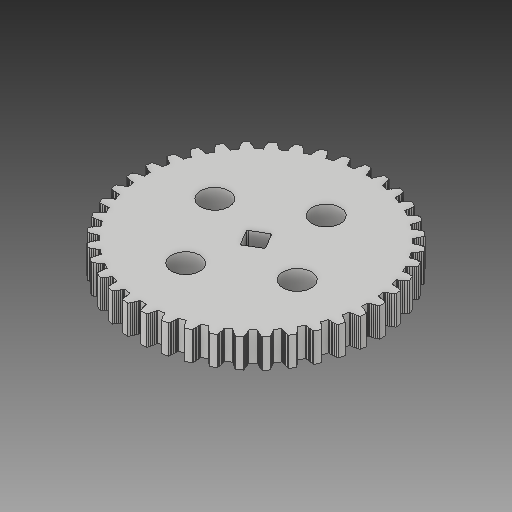
# Autodesk Inventor part: gear40
Saved by Autodesk Inventor 2019 (Build 230136000, 136)
## iProperties
Created: 2018-12-28
Part Number: gear40
Material: Generic
Document SubType Name: Modeling
Designer: Varga Daniel
Density: 1 g/cm^3
Appearance: Default
Sending System: SolidWorks 2018
Last Author: david
Last Saved: 2018-12-28
Author: Varga Daniel
Autodesk Inventor part; units mm, degrees
ref_plane "YZ Plane" through (0, 0, 0) normal (1, 0, 0) x (0, 1, 0)
ref_plane "XZ Plane" through (0, 0, 0) normal (0, 1, 0) x (-1, 0, 0)
ref_plane "XY Plane" through (0, 0, 0) normal (0, 0, 1) x (1, 0, 0)
sketch "Sketch5" plane through (0, 0, 0) normal (0, 1, 0) x (-1, 0, 0)
  line L0 (1.6245, 18.6336) -> (1.5605, 18.6409)
  line L1 (1.5605, 18.6409) -> (1.4964, 18.6492)
  line L2 (1.4964, 18.6492) -> (1.3679, 18.6686)
  line L3 (1.3679, 18.6686) -> (1.1102, 18.7172)
  line L4 (1.1102, 18.7172) -> (0.8515, 18.7777)
  line L5 (0.8515, 18.7777) -> (0.5922, 18.8492)
  line L6 (0.5922, 18.8492) -> (0.3324, 18.931)
  line L7 (0.3324, 18.931) -> (0.0723, 19.0226)
  line L8 (0.0723, 19.0226) -> (0.0134, 20.0093)
  line L9 (0.0134, 20.0093) -> (0.2607, 20.1312)
  line L10 (0.2607, 20.1312) -> (0.5089, 20.2434)
  line L11 (0.5089, 20.2434) -> (0.7578, 20.3453)
  line L12 (0.7578, 20.3453) -> (1.0074, 20.4362)
  line L13 (1.0074, 20.4362) -> (1.2576, 20.5151)
  line L14 (1.2576, 20.5151) -> (1.3828, 20.5496)
  line L15 (1.3828, 20.5496) -> (1.4455, 20.5655)
  line L16 (1.4455, 20.5655) -> (1.5081, 20.5804)
  line L17 (1.5081, 20.5804) -> (1.5283, 21.6521)
  line L18 (1.5283, 21.6521) -> (1.4663, 21.6694)
  line L19 (1.4663, 21.6694) -> (1.4042, 21.6877)
  line L20 (1.4042, 21.6877) -> (1.2804, 21.7268)
  line L21 (1.2804, 21.7268) -> (1.0334, 21.8151)
  line L22 (1.0334, 21.8151) -> (0.7874, 21.9154)
  line L23 (0.7874, 21.9154) -> (0.5425, 22.0266)
  line L24 (0.5425, 22.0266) -> (0.2987, 22.1481)
  line L25 (0.2987, 22.1481) -> (0.0561, 22.2792)
  line L26 (0.0561, 22.2792) -> (0.1523, 23.263)
  line L27 (0.1523, 23.263) -> (0.4156, 23.3447)
  line L28 (0.4156, 23.3447) -> (0.6783, 23.4167)
  line L29 (0.6783, 23.4167) -> (0.9401, 23.4783)
  line L30 (0.9401, 23.4783) -> (1.2009, 23.5291)
  line L31 (1.2009, 23.5291) -> (1.4603, 23.5679)
  line L32 (1.4603, 23.5679) -> (1.5894, 23.5824)
  line L33 (1.5894, 23.5824) -> (1.6537, 23.5883)
  line L34 (1.6537, 23.5883) -> (1.718, 23.5932)
  line L35 (1.718, 23.5932) -> (1.9056, 24.6486)
  line L36 (1.9056, 24.6486) -> (1.847, 24.6754)
  line L37 (1.847, 24.6754) -> (1.7886, 24.7031)
  line L38 (1.7886, 24.7031) -> (1.6724, 24.7612)
  line L39 (1.6724, 24.7612) -> (1.4423, 24.887)
  line L40 (1.4423, 24.887) -> (1.215, 25.0245)
  line L41 (1.215, 25.0245) -> (0.9905, 25.1727)
  line L42 (0.9905, 25.1727) -> (0.7687, 25.3308)
  line L43 (0.7687, 25.3308) -> (0.5496, 25.4982)
  line L44 (0.5496, 25.4982) -> (0.7984, 26.4549)
  line L45 (0.7984, 26.4549) -> (1.0713, 26.4944)
  line L46 (1.0713, 26.4944) -> (1.342, 26.5244)
  line L47 (1.342, 26.5244) -> (1.6103, 26.5443)
  line L48 (1.6103, 26.5443) -> (1.8758, 26.5537)
  line L49 (1.8758, 26.5537) -> (2.1381, 26.5514)
  line L50 (2.1381, 26.5514) -> (2.2678, 26.5455)
  line L51 (2.2678, 26.5455) -> (2.3323, 26.5413)
  line L52 (2.3323, 26.5413) -> (2.3965, 26.5361)
  line L53 (2.3965, 26.5361) -> (2.7469, 27.5491)
  line L54 (2.7469, 27.5491) -> (2.6932, 27.5847)
  line L55 (2.6932, 27.5847) -> (2.6399, 27.6213)
  line L56 (2.6399, 27.6213) -> (2.5342, 27.6968)
  line L57 (2.5342, 27.6968) -> (2.3266, 27.8571)
  line L58 (2.3266, 27.8571) -> (2.1237, 28.0284)
  line L59 (2.1237, 28.0284) -> (1.9251, 28.2099)
  line L60 (1.9251, 28.2099) -> (1.7307, 28.4007)
  line L61 (1.7307, 28.4007) -> (1.5406, 28.6004)
  line L62 (1.5406, 28.6004) -> (1.936, 29.5064)
  line L63 (1.936, 29.5064) -> (2.2117, 29.5027)
  line L64 (2.2117, 29.5027) -> (2.4838, 29.49)
  line L65 (2.4838, 29.49) -> (2.7519, 29.4677)
  line L66 (2.7519, 29.4677) -> (3.0155, 29.4354)
  line L67 (3.0155, 29.4354) -> (3.2742, 29.3922)
  line L68 (3.2742, 29.3922) -> (3.4015, 29.3661)
  line L69 (3.4015, 29.3661) -> (3.4645, 29.3518)
  line L70 (3.4645, 29.3518) -> (3.5271, 29.3366)
  line L71 (3.5271, 29.3366) -> (4.0316, 30.2823)
  line L72 (4.0316, 30.2823) -> (3.9842, 30.3259)
  line L73 (3.9842, 30.3259) -> (3.9372, 30.3703)
  line L74 (3.9372, 30.3703) -> (3.8447, 30.4614)
  line L75 (3.8447, 30.4614) -> (3.6647, 30.6522)
  line L76 (3.6647, 30.6522) -> (3.491, 30.8533)
  line L77 (3.491, 30.8533) -> (3.3233, 31.0636)
  line L78 (3.3233, 31.0636) -> (3.1612, 31.2824)
  line L79 (3.1612, 31.2824) -> (3.0046, 31.5094)
  line L80 (3.0046, 31.5094) -> (3.5369, 32.3423)
  line L81 (3.5369, 32.3423) -> (3.8086, 32.2956)
  line L82 (3.8086, 32.2956) -> (4.0754, 32.2404)
  line L83 (4.0754, 32.2404) -> (4.3367, 32.1765)
  line L84 (4.3367, 32.1765) -> (4.592, 32.1034)
  line L85 (4.592, 32.1034) -> (4.8408, 32.0202)
  line L86 (4.8408, 32.0202) -> (4.9624, 31.9745)
  line L87 (4.9624, 31.9745) -> (5.0224, 31.9505)
  line L88 (5.0224, 31.9505) -> (5.0819, 31.9258)
  line L89 (5.0819, 31.9258) -> (5.7281, 32.7809)
  line L90 (5.7281, 32.7809) -> (5.6881, 32.8314)
  line L91 (5.6881, 32.8314) -> (5.6487, 32.8826)
  line L92 (5.6487, 32.8826) -> (5.5715, 32.9871)
  line L93 (5.5715, 32.9871) -> (5.4236, 33.2037)
  line L94 (5.4236, 33.2037) -> (5.2835, 33.4294)
  line L95 (5.2835, 33.4294) -> (5.1507, 33.6633)
  line L96 (5.1507, 33.6633) -> (5.0248, 33.9049)
  line L97 (5.0248, 33.9049) -> (4.9057, 34.1535)
  line L98 (4.9057, 34.1535) -> (5.5617, 34.893)
  line L99 (5.5617, 34.893) -> (5.8228, 34.8043)
  line L100 (5.8228, 34.8043) -> (6.0776, 34.7081)
  line L101 (6.0776, 34.7081) -> (6.3257, 34.6041)
  line L102 (6.3257, 34.6041) -> (6.5665, 34.4919)
  line L103 (6.5665, 34.4919) -> (6.7992, 34.3708)
  line L104 (6.7992, 34.3708) -> (6.9121, 34.3067)
  line L105 (6.9121, 34.3067) -> (6.9677, 34.2736)
  line L106 (6.9677, 34.2736) -> (7.0225, 34.2398)
  line L107 (7.0225, 34.2398) -> (7.7946, 34.9834)
  line L108 (7.7946, 34.9834) -> (7.7629, 35.0395)
  line L109 (7.7629, 35.0395) -> (7.732, 35.0962)
  line L110 (7.732, 35.0962) -> (7.6721, 35.2115)
  line L111 (7.6721, 35.2115) -> (7.5599, 35.4486)
  line L112 (7.5599, 35.4486) -> (7.4569, 35.6934)
  line L113 (7.4569, 35.6934) -> (7.3623, 35.9452)
  line L114 (7.3623, 35.9452) -> (7.2758, 36.2035)
  line L115 (7.2758, 36.2035) -> (7.197, 36.4677)
  line L116 (7.197, 36.4677) -> (7.9606, 37.0954)
  line L117 (7.9606, 37.0954) -> (8.2046, 36.967)
  line L118 (8.2046, 36.967) -> (8.4412, 36.8321)
  line L119 (8.4412, 36.8321) -> (8.67, 36.6906)
  line L120 (8.67, 36.6906) -> (8.8903, 36.5421)
  line L121 (8.8903, 36.5421) -> (9.1012, 36.3861)
  line L122 (9.1012, 36.3861) -> (9.2027, 36.3051)
  line L123 (9.2027, 36.3051) -> (9.2524, 36.2638)
  line L124 (9.2524, 36.2638) -> (9.3013, 36.2218)
  line L125 (9.3013, 36.2218) -> (10.1802, 36.8354)
  line L126 (10.1802, 36.8354) -> (10.1577, 36.8958)
  line L127 (10.1577, 36.8958) -> (10.136, 36.9567)
  line L128 (10.136, 36.9567) -> (10.0949, 37.0799)
  line L129 (10.0949, 37.0799) -> (10.0212, 37.3316)
  line L130 (10.0212, 37.3316) -> (9.9577, 37.5896)
  line L131 (9.9577, 37.5896) -> (9.9037, 37.8531)
  line L132 (9.9037, 37.8531) -> (9.8586, 38.1217)
  line L133 (9.8586, 38.1217) -> (9.8221, 38.395)
  line L134 (9.8221, 38.395) -> (10.6746, 38.8955)
  line L135 (10.6746, 38.8955) -> (10.8954, 38.7305)
  line L136 (10.8954, 38.7305) -> (11.1081, 38.5603)
  line L137 (11.1081, 38.5603) -> (11.3119, 38.3847)
  line L138 (11.3119, 38.3847) -> (11.5062, 38.2036)
  line L139 (11.5062, 38.2036) -> (11.6901, 38.0165)
  line L140 (11.6901, 38.0165) -> (11.7777, 37.9206)
  line L141 (11.7777, 37.9206) -> (11.8203, 37.872)
  line L142 (11.8203, 37.872) -> (11.862, 37.823)
  line L143 (11.862, 37.823) -> (12.8261, 38.2915)
  line L144 (12.8261, 38.2915) -> (12.8133, 38.3546)
  line L145 (12.8133, 38.3546) -> (12.8014, 38.4182)
  line L146 (12.8014, 38.4182) -> (12.7801, 38.5463)
  line L147 (12.7801, 38.5463) -> (12.7467, 38.8064)
  line L148 (12.7467, 38.8064) -> (12.7243, 39.0711)
  line L149 (12.7243, 39.0711) -> (12.7122, 39.3399)
  line L150 (12.7122, 39.3399) -> (12.7097, 39.6122)
  line L151 (12.7097, 39.6122) -> (12.7164, 39.8879)
  line L152 (12.7164, 39.8879) -> (13.6367, 40.2489)
  line L153 (13.6367, 40.2489) -> (13.829, 40.0513)
  line L154 (13.829, 40.0513) -> (14.0124, 39.8499)
  line L155 (14.0124, 39.8499) -> (14.1862, 39.6447)
  line L156 (14.1862, 39.6447) -> (14.3498, 39.4354)
  line L157 (14.3498, 39.4354) -> (14.5022, 39.2219)
  line L158 (14.5022, 39.2219) -> (14.5737, 39.1134)
  line L159 (14.5737, 39.1134) -> (14.6082, 39.0587)
  line L160 (14.6082, 39.0587) -> (14.6417, 39.0038)
  line L161 (14.6417, 39.0038) -> (15.6672, 39.3157)
  line L162 (15.6672, 39.3157) -> (15.6645, 39.3801)
  line L163 (15.6645, 39.3801) -> (15.6627, 39.4447)
  line L164 (15.6627, 39.4447) -> (15.6617, 39.5746)
  line L165 (15.6617, 39.5746) -> (15.6693, 39.8368)
  line L166 (15.6693, 39.8368) -> (15.6886, 40.1017)
  line L167 (15.6886, 40.1017) -> (15.7187, 40.369)
  line L168 (15.7187, 40.369) -> (15.7589, 40.6384)
  line L169 (15.7589, 40.6384) -> (15.8086, 40.9096)
  line L170 (15.8086, 40.9096) -> (16.774, 41.1222)
  line L171 (16.774, 41.1222) -> (16.9331, 40.897)
  line L172 (16.9331, 40.897) -> (17.0827, 40.6694)
  line L173 (17.0827, 40.6694) -> (17.2223, 40.4394)
  line L174 (17.2223, 40.4394) -> (17.3511, 40.2071)
  line L175 (17.3511, 40.2071) -> (17.4682, 39.9724)
  line L176 (17.4682, 39.9724) -> (17.5219, 39.8541)
  line L177 (17.5219, 39.8541) -> (17.5474, 39.7948)
  line L178 (17.5474, 39.7948) -> (17.5719, 39.7352)
  line L179 (17.5719, 39.7352) -> (18.6336, 39.8829)
  line L180 (18.6336, 39.8829) -> (18.6409, 39.9469)
  line L181 (18.6409, 39.9469) -> (18.6493, 40.011)
  line L182 (18.6493, 40.011) -> (18.6686, 40.1394)
  line L183 (18.6686, 40.1394) -> (18.7172, 40.3972)
  line L184 (18.7172, 40.3972) -> (18.7777, 40.6558)
  line L185 (18.7777, 40.6558) -> (18.8492, 40.9152)
  line L186 (18.8492, 40.9152) -> (18.931, 41.175)
  line L187 (18.931, 41.175) -> (19.0226, 41.435)
  line L188 (19.0226, 41.435) -> (20.0093, 41.494)
  line L189 (20.0093, 41.494) -> (20.1312, 41.2467)
  line L190 (20.1312, 41.2467) -> (20.2434, 40.9985)
  line L191 (20.2434, 40.9985) -> (20.3453, 40.7495)
  line L192 (20.3453, 40.7495) -> (20.4362, 40.4999)
  line L193 (20.4362, 40.4999) -> (20.5151, 40.2498)
  line L194 (20.5151, 40.2498) -> (20.5496, 40.1246)
  line L195 (20.5496, 40.1246) -> (20.5655, 40.0619)
  line L196 (20.5655, 40.0619) -> (20.5804, 39.9993)
  line L197 (20.5804, 39.9993) -> (21.6521, 39.9791)
  line L198 (21.6521, 39.9791) -> (21.6694, 40.0411)
  line L199 (21.6694, 40.0411) -> (21.6877, 40.1031)
  line L200 (21.6877, 40.1031) -> (21.7269, 40.227)
  line L201 (21.7269, 40.227) -> (21.8151, 40.4739)
  line L202 (21.8151, 40.4739) -> (21.9154, 40.7199)
  line L203 (21.9154, 40.7199) -> (22.0266, 40.9649)
  line L204 (22.0266, 40.9649) -> (22.148, 41.2087)
  line L205 (22.148, 41.2087) -> (22.2792, 41.4512)
  line L206 (22.2792, 41.4512) -> (23.263, 41.3551)
  line L207 (23.263, 41.3551) -> (23.3447, 41.0918)
  line L208 (23.3447, 41.0918) -> (23.4167, 40.8291)
  line L209 (23.4167, 40.8291) -> (23.4783, 40.5672)
  line L210 (23.4783, 40.5672) -> (23.5291, 40.3065)
  line L211 (23.5291, 40.3065) -> (23.5679, 40.0471)
  line L212 (23.5679, 40.0471) -> (23.5824, 39.918)
  line L213 (23.5824, 39.918) -> (23.5883, 39.8536)
  line L214 (23.5883, 39.8536) -> (23.5932, 39.7894)
  line L215 (23.5932, 39.7894) -> (24.6486, 39.6018)
  line L216 (24.6486, 39.6018) -> (24.6754, 39.6604)
  line L217 (24.6754, 39.6604) -> (24.7031, 39.7188)
  line L218 (24.7031, 39.7188) -> (24.7612, 39.8349)
  line L219 (24.7612, 39.8349) -> (24.887, 40.0651)
  line L220 (24.887, 40.0651) -> (25.0245, 40.2924)
  line L221 (25.0245, 40.2924) -> (25.1727, 40.5169)
  line L222 (25.1727, 40.5169) -> (25.3307, 40.7387)
  line L223 (25.3307, 40.7387) -> (25.4982, 40.9577)
  line L224 (25.4982, 40.9577) -> (26.4549, 40.7089)
  line L225 (26.4549, 40.7089) -> (26.4944, 40.436)
  line L226 (26.4944, 40.436) -> (26.5243, 40.1653)
  line L227 (26.5243, 40.1653) -> (26.5443, 39.8971)
  line L228 (26.5443, 39.8971) -> (26.5537, 39.6316)
  line L229 (26.5537, 39.6316) -> (26.5514, 39.3693)
  line L230 (26.5514, 39.3693) -> (26.5455, 39.2395)
  line L231 (26.5455, 39.2395) -> (26.5413, 39.175)
  line L232 (26.5413, 39.175) -> (26.5361, 39.1108)
  line L233 (26.5361, 39.1108) -> (27.5491, 38.7604)
  line L234 (27.5491, 38.7604) -> (27.5847, 38.8141)
  line L235 (27.5847, 38.8141) -> (27.6212, 38.8675)
  line L236 (27.6212, 38.8675) -> (27.6968, 38.9731)
  line L237 (27.6968, 38.9731) -> (27.8571, 39.1807)
  line L238 (27.8571, 39.1807) -> (28.0284, 39.3837)
  line L239 (28.0284, 39.3837) -> (28.2099, 39.5823)
  line L240 (28.2099, 39.5823) -> (28.4007, 39.7766)
  line L241 (28.4007, 39.7766) -> (28.6004, 39.9668)
  line L242 (28.6004, 39.9668) -> (29.5064, 39.5714)
  line L243 (29.5064, 39.5714) -> (29.5027, 39.2957)
  line L244 (29.5027, 39.2957) -> (29.4899, 39.0236)
  line L245 (29.4899, 39.0236) -> (29.4677, 38.7555)
  line L246 (29.4677, 38.7555) -> (29.4354, 38.4918)
  line L247 (29.4354, 38.4918) -> (29.3922, 38.2331)
  line L248 (29.3922, 38.2331) -> (29.366, 38.1059)
  line L249 (29.366, 38.1059) -> (29.3518, 38.0429)
  line L250 (29.3518, 38.0429) -> (29.3366, 37.9802)
  line L251 (29.3366, 37.9802) -> (30.2823, 37.4757)
  line L252 (30.2823, 37.4757) -> (30.3259, 37.5231)
  line L253 (30.3259, 37.5231) -> (30.3704, 37.5702)
  line L254 (30.3704, 37.5702) -> (30.4615, 37.6628)
  line L255 (30.4615, 37.6628) -> (30.6523, 37.8427)
  line L256 (30.6523, 37.8427) -> (30.8533, 38.0164)
  line L257 (30.8533, 38.0164) -> (31.0636, 38.1842)
  line L258 (31.0636, 38.1842) -> (31.2825, 38.3463)
  line L259 (31.2825, 38.3463) -> (31.5095, 38.5028)
  line L260 (31.5095, 38.5028) -> (32.3424, 37.9706)
  line L261 (32.3424, 37.9706) -> (32.2956, 37.6988)
  line L262 (32.2956, 37.6988) -> (32.2405, 37.4321)
  line L263 (32.2405, 37.4321) -> (32.1766, 37.1708)
  line L264 (32.1766, 37.1708) -> (32.1035, 36.9154)
  line L265 (32.1035, 36.9154) -> (32.0203, 36.6667)
  line L266 (32.0203, 36.6667) -> (31.9746, 36.5451)
  line L267 (31.9746, 36.5451) -> (31.9506, 36.4851)
  line L268 (31.9506, 36.4851) -> (31.9259, 36.4256)
  line L269 (31.9259, 36.4256) -> (32.781, 35.7793)
  line L270 (32.781, 35.7793) -> (32.8315, 35.8194)
  line L271 (32.8315, 35.8194) -> (32.8827, 35.8588)
  line L272 (32.8827, 35.8588) -> (32.9872, 35.936)
  line L273 (32.9872, 35.936) -> (33.2038, 36.0839)
  line L274 (33.2038, 36.0839) -> (33.4295, 36.224)
  line L275 (33.4295, 36.224) -> (33.6634, 36.3567)
  line L276 (33.6634, 36.3567) -> (33.905, 36.4826)
  line L277 (33.905, 36.4826) -> (34.1536, 36.6018)
  line L278 (34.1536, 36.6018) -> (34.893, 35.9457)
  line L279 (34.893, 35.9457) -> (34.8044, 35.6847)
  line L280 (34.8044, 35.6847) -> (34.7082, 35.4298)
  line L281 (34.7082, 35.4298) -> (34.6042, 35.1817)
  line L282 (34.6042, 35.1817) -> (34.492, 34.941)
  line L283 (34.492, 34.941) -> (34.3709, 34.7083)
  line L284 (34.3709, 34.7083) -> (34.3067, 34.5953)
  line L285 (34.3067, 34.5953) -> (34.2737, 34.5398)
  line L286 (34.2737, 34.5398) -> (34.2399, 34.4849)
  line L287 (34.2399, 34.4849) -> (34.9834, 33.7128)
  line L288 (34.9834, 33.7128) -> (35.0395, 33.7445)
  line L289 (35.0395, 33.7445) -> (35.0963, 33.7754)
  line L290 (35.0963, 33.7754) -> (35.2116, 33.8353)
  line L291 (35.2116, 33.8353) -> (35.4486, 33.9475)
  line L292 (35.4486, 33.9475) -> (35.6935, 34.0506)
  line L293 (35.6935, 34.0506) -> (35.9453, 34.1451)
  line L294 (35.9453, 34.1451) -> (36.2036, 34.2316)
  line L295 (36.2036, 34.2316) -> (36.4678, 34.3104)
  line L296 (36.4678, 34.3104) -> (37.0955, 33.5468)
  line L297 (37.0955, 33.5468) -> (36.9671, 33.3028)
  line L298 (36.9671, 33.3028) -> (36.8322, 33.0662)
  line L299 (36.8322, 33.0662) -> (36.6907, 32.8374)
  line L300 (36.6907, 32.8374) -> (36.5422, 32.6171)
  line L301 (36.5422, 32.6171) -> (36.3862, 32.4063)
  line L302 (36.3862, 32.4063) -> (36.3052, 32.3048)
  line L303 (36.3052, 32.3048) -> (36.2638, 32.2551)
  line L304 (36.2638, 32.2551) -> (36.2219, 32.2062)
  line L305 (36.2219, 32.2062) -> (36.8355, 31.3273)
  line L306 (36.8355, 31.3273) -> (36.8959, 31.3498)
  line L307 (36.8959, 31.3498) -> (36.9568, 31.3715)
  line L308 (36.9568, 31.3715) -> (37.08, 31.4125)
  line L309 (37.08, 31.4125) -> (37.3317, 31.4863)
  line L310 (37.3317, 31.4863) -> (37.5896, 31.5498)
  line L311 (37.5896, 31.5498) -> (37.8532, 31.6038)
  line L312 (37.8532, 31.6038) -> (38.1218, 31.6488)
  line L313 (38.1218, 31.6488) -> (38.3951, 31.6853)
  line L314 (38.3951, 31.6853) -> (38.8956, 30.8329)
  line L315 (38.8956, 30.8329) -> (38.7306, 30.612)
  line L316 (38.7306, 30.612) -> (38.5603, 30.3994)
  line L317 (38.5603, 30.3994) -> (38.3848, 30.1956)
  line L318 (38.3848, 30.1956) -> (38.2037, 30.0012)
  line L319 (38.2037, 30.0012) -> (38.0166, 29.8174)
  line L320 (38.0166, 29.8174) -> (37.9207, 29.7298)
  line L321 (37.9207, 29.7298) -> (37.8721, 29.6872)
  line L322 (37.8721, 29.6872) -> (37.823, 29.6454)
  line L323 (37.823, 29.6454) -> (38.2916, 28.6814)
  line L324 (38.2916, 28.6814) -> (38.3547, 28.6941)
  line L325 (38.3547, 28.6941) -> (38.4183, 28.706)
  line L326 (38.4183, 28.706) -> (38.5464, 28.7273)
  line L327 (38.5464, 28.7273) -> (38.8065, 28.7608)
  line L328 (38.8065, 28.7608) -> (39.0712, 28.7831)
  line L329 (39.0712, 28.7831) -> (39.34, 28.7953)
  line L330 (39.34, 28.7953) -> (39.6123, 28.7977)
  line L331 (39.6123, 28.7977) -> (39.888, 28.791)
  line L332 (39.888, 28.791) -> (40.249, 27.8708)
  line L333 (40.249, 27.8708) -> (40.0514, 27.6784)
  line L334 (40.0514, 27.6784) -> (39.85, 27.4951)
  line L335 (39.85, 27.4951) -> (39.6447, 27.3212)
  line L336 (39.6447, 27.3212) -> (39.4354, 27.1576)
  line L337 (39.4354, 27.1576) -> (39.2219, 27.0053)
  line L338 (39.2219, 27.0053) -> (39.1135, 26.9338)
  line L339 (39.1135, 26.9338) -> (39.0588, 26.8993)
  line L340 (39.0588, 26.8993) -> (39.0038, 26.8657)
  line L341 (39.0038, 26.8657) -> (39.3158, 25.8402)
  line L342 (39.3158, 25.8402) -> (39.3802, 25.843)
  line L343 (39.3802, 25.843) -> (39.4448, 25.8448)
  line L344 (39.4448, 25.8448) -> (39.5747, 25.8458)
  line L345 (39.5747, 25.8458) -> (39.8368, 25.8382)
  line L346 (39.8368, 25.8382) -> (40.1018, 25.8188)
  line L347 (40.1018, 25.8188) -> (40.3691, 25.7887)
  line L348 (40.3691, 25.7887) -> (40.6385, 25.7486)
  line L349 (40.6385, 25.7486) -> (40.9097, 25.6988)
  line L350 (40.9097, 25.6988) -> (41.1223, 24.7334)
  line L351 (41.1223, 24.7334) -> (40.897, 24.5742)
  line L352 (40.897, 24.5742) -> (40.6693, 24.4246)
  line L353 (40.6693, 24.4246) -> (40.4394, 24.285)
  line L354 (40.4394, 24.285) -> (40.2071, 24.1561)
  line L355 (40.2071, 24.1561) -> (39.9723, 24.0391)
  line L356 (39.9723, 24.0391) -> (39.8541, 23.9854)
  line L357 (39.8541, 23.9854) -> (39.7947, 23.9599)
  line L358 (39.7947, 23.9599) -> (39.7351, 23.9354)
  line L359 (39.7351, 23.9354) -> (39.8828, 22.8737)
  line L360 (39.8828, 22.8737) -> (39.9468, 22.8664)
  line L361 (39.9468, 22.8664) -> (40.0109, 22.858)
  line L362 (40.0109, 22.858) -> (40.1393, 22.8387)
  line L363 (40.1393, 22.8387) -> (40.3971, 22.7901)
  line L364 (40.3971, 22.7901) -> (40.6558, 22.7296)
  line L365 (40.6558, 22.7296) -> (40.9151, 22.6581)
  line L366 (40.9151, 22.6581) -> (41.1749, 22.5763)
  line L367 (41.1749, 22.5763) -> (41.435, 22.4847)
  line L368 (41.435, 22.4847) -> (41.4939, 21.498)
  line L369 (41.4939, 21.498) -> (41.2466, 21.3761)
  line L370 (41.2466, 21.3761) -> (40.9984, 21.2639)
  line L371 (40.9984, 21.2639) -> (40.7494, 21.162)
  line L372 (40.7494, 21.162) -> (40.4998, 21.0711)
  line L373 (40.4998, 21.0711) -> (40.2497, 20.9922)
  line L374 (40.2497, 20.9922) -> (40.1245, 20.9577)
  line L375 (40.1245, 20.9577) -> (40.0618, 20.9418)
  line L376 (40.0618, 20.9418) -> (39.9991, 20.9268)
  line L377 (39.9991, 20.9268) -> (39.9789, 19.8552)
  line L378 (39.9789, 19.8552) -> (40.041, 19.8379)
  line L379 (40.041, 19.8379) -> (40.103, 19.8196)
  line L380 (40.103, 19.8196) -> (40.2268, 19.7804)
  line L381 (40.2268, 19.7804) -> (40.4738, 19.6922)
  line L382 (40.4738, 19.6922) -> (40.7198, 19.5919)
  line L383 (40.7198, 19.5919) -> (40.9647, 19.4807)
  line L384 (40.9647, 19.4807) -> (41.2085, 19.3592)
  line L385 (41.2085, 19.3592) -> (41.4511, 19.2281)
  line L386 (41.4511, 19.2281) -> (41.355, 18.2443)
  line L387 (41.355, 18.2443) -> (41.0918, 18.1626)
  line L388 (41.0918, 18.1626) -> (40.8291, 18.0907)
  line L389 (40.8291, 18.0907) -> (40.5673, 18.029)
  line L390 (40.5673, 18.029) -> (40.3066, 17.9782)
  line L391 (40.3066, 17.9782) -> (40.0472, 17.9394)
  line L392 (40.0472, 17.9394) -> (39.9181, 17.9249)
  line L393 (39.9181, 17.9249) -> (39.8537, 17.919)
  line L394 (39.8537, 17.919) -> (39.7895, 17.9141)
  line L395 (39.7895, 17.9141) -> (39.6018, 16.8587)
  line L396 (39.6018, 16.8587) -> (39.6604, 16.832)
  line L397 (39.6604, 16.832) -> (39.7188, 16.8042)
  line L398 (39.7188, 16.8042) -> (39.835, 16.7462)
  line L399 (39.835, 16.7462) -> (40.0651, 16.6203)
  line L400 (40.0651, 16.6203) -> (40.2924, 16.4828)
  line L401 (40.2924, 16.4828) -> (40.517, 16.3346)
  line L402 (40.517, 16.3346) -> (40.7388, 16.1766)
  line L403 (40.7388, 16.1766) -> (40.9578, 16.0091)
  line L404 (40.9578, 16.0091) -> (40.709, 15.0524)
  line L405 (40.709, 15.0524) -> (40.4361, 15.0129)
  line L406 (40.4361, 15.0129) -> (40.1654, 14.983)
  line L407 (40.1654, 14.983) -> (39.8971, 14.963)
  line L408 (39.8971, 14.963) -> (39.6316, 14.9536)
  line L409 (39.6316, 14.9536) -> (39.3694, 14.9559)
  line L410 (39.3694, 14.9559) -> (39.2396, 14.9618)
  line L411 (39.2396, 14.9618) -> (39.1751, 14.966)
  line L412 (39.1751, 14.966) -> (39.1109, 14.9712)
  line L413 (39.1109, 14.9712) -> (38.7605, 13.9582)
  line L414 (38.7605, 13.9582) -> (38.8142, 13.9226)
  line L415 (38.8142, 13.9226) -> (38.8675, 13.886)
  line L416 (38.8675, 13.886) -> (38.9732, 13.8105)
  line L417 (38.9732, 13.8105) -> (39.1808, 13.6502)
  line L418 (39.1808, 13.6502) -> (39.3838, 13.4788)
  line L419 (39.3838, 13.4788) -> (39.5823, 13.2974)
  line L420 (39.5823, 13.2974) -> (39.7767, 13.1066)
  line L421 (39.7767, 13.1066) -> (39.9668, 12.9069)
  line L422 (39.9668, 12.9069) -> (39.5714, 12.0009)
  line L423 (39.5714, 12.0009) -> (39.2957, 12.0046)
  line L424 (39.2957, 12.0046) -> (39.0236, 12.0173)
  line L425 (39.0236, 12.0173) -> (38.7555, 12.0396)
  line L426 (38.7555, 12.0396) -> (38.4919, 12.0719)
  line L427 (38.4919, 12.0719) -> (38.2332, 12.1151)
  line L428 (38.2332, 12.1151) -> (38.1059, 12.1412)
  line L429 (38.1059, 12.1412) -> (38.0429, 12.1555)
  line L430 (38.0429, 12.1555) -> (37.9803, 12.1707)
  line L431 (37.9803, 12.1707) -> (37.4757, 11.225)
  line L432 (37.4757, 11.225) -> (37.5232, 11.1814)
  line L433 (37.5232, 11.1814) -> (37.5702, 11.137)
  line L434 (37.5702, 11.137) -> (37.6627, 11.0458)
  line L435 (37.6627, 11.0458) -> (37.8427, 10.8551)
  line L436 (37.8427, 10.8551) -> (38.0164, 10.654)
  line L437 (38.0164, 10.654) -> (38.1841, 10.4438)
  line L438 (38.1841, 10.4438) -> (38.3462, 10.2249)
  line L439 (38.3462, 10.2249) -> (38.5028, 9.9979)
  line L440 (38.5028, 9.9979) -> (37.9705, 9.165)
  line L441 (37.9705, 9.165) -> (37.6988, 9.2117)
  line L442 (37.6988, 9.2117) -> (37.432, 9.2669)
  line L443 (37.432, 9.2669) -> (37.1707, 9.3308)
  line L444 (37.1707, 9.3308) -> (36.9154, 9.4039)
  line L445 (36.9154, 9.4039) -> (36.6666, 9.4871)
  line L446 (36.6666, 9.4871) -> (36.545, 9.5328)
  line L447 (36.545, 9.5328) -> (36.485, 9.5568)
  line L448 (36.485, 9.5568) -> (36.4255, 9.5815)
  line L449 (36.4255, 9.5815) -> (35.7792, 8.7264)
  line L450 (35.7792, 8.7264) -> (35.8193, 8.6759)
  line L451 (35.8193, 8.6759) -> (35.8587, 8.6247)
  line L452 (35.8587, 8.6247) -> (35.9359, 8.5202)
  line L453 (35.9359, 8.5202) -> (36.0838, 8.3036)
  line L454 (36.0838, 8.3036) -> (36.2239, 8.0779)
  line L455 (36.2239, 8.0779) -> (36.3567, 7.844)
  line L456 (36.3567, 7.844) -> (36.4825, 7.6024)
  line L457 (36.4825, 7.6024) -> (36.6017, 7.3538)
  line L458 (36.6017, 7.3538) -> (35.9456, 6.6144)
  line L459 (35.9456, 6.6144) -> (35.6846, 6.703)
  line L460 (35.6846, 6.703) -> (35.4298, 6.7992)
  line L461 (35.4298, 6.7992) -> (35.1817, 6.9032)
  line L462 (35.1817, 6.9032) -> (34.9409, 7.0154)
  line L463 (34.9409, 7.0154) -> (34.7082, 7.1365)
  line L464 (34.7082, 7.1365) -> (34.5953, 7.2007)
  line L465 (34.5953, 7.2007) -> (34.5397, 7.2337)
  line L466 (34.5397, 7.2337) -> (34.4849, 7.2675)
  line L467 (34.4849, 7.2675) -> (33.7128, 6.5239)
  line L468 (33.7128, 6.5239) -> (33.7444, 6.4678)
  line L469 (33.7444, 6.4678) -> (33.7754, 6.4111)
  line L470 (33.7754, 6.4111) -> (33.8352, 6.2958)
  line L471 (33.8352, 6.2958) -> (33.9474, 6.0587)
  line L472 (33.9474, 6.0587) -> (34.0505, 5.8139)
  line L473 (34.0505, 5.8139) -> (34.145, 5.5621)
  line L474 (34.145, 5.5621) -> (34.2316, 5.3038)
  line L475 (34.2316, 5.3038) -> (34.3103, 5.0396)
  line L476 (34.3103, 5.0396) -> (33.5467, 4.4119)
  line L477 (33.5467, 4.4119) -> (33.3027, 4.5403)
  line L478 (33.3027, 4.5403) -> (33.0661, 4.6752)
  line L479 (33.0661, 4.6752) -> (32.8373, 4.8167)
  line L480 (32.8373, 4.8167) -> (32.6171, 4.9652)
  line L481 (32.6171, 4.9652) -> (32.4062, 5.1212)
  line L482 (32.4062, 5.1212) -> (32.3047, 5.2022)
  line L483 (32.3047, 5.2022) -> (32.255, 5.2436)
  line L484 (32.255, 5.2436) -> (32.206, 5.2855)
  line L485 (32.206, 5.2855) -> (31.3272, 4.6719)
  line L486 (31.3272, 4.6719) -> (31.3497, 4.6115)
  line L487 (31.3497, 4.6115) -> (31.3713, 4.5507)
  line L488 (31.3713, 4.5507) -> (31.4124, 4.4274)
  line L489 (31.4124, 4.4274) -> (31.4862, 4.1757)
  line L490 (31.4862, 4.1757) -> (31.5496, 3.9178)
  line L491 (31.5496, 3.9178) -> (31.6037, 3.6543)
  line L492 (31.6037, 3.6543) -> (31.6487, 3.3856)
  line L493 (31.6487, 3.3856) -> (31.6852, 3.1123)
  line L494 (31.6852, 3.1123) -> (30.8328, 2.6118)
  line L495 (30.8328, 2.6118) -> (30.6119, 2.7769)
  line L496 (30.6119, 2.7769) -> (30.3993, 2.9471)
  line L497 (30.3993, 2.9471) -> (30.1954, 3.1226)
  line L498 (30.1954, 3.1226) -> (30.0011, 3.3038)
  line L499 (30.0011, 3.3038) -> (29.8172, 3.4908)
  line L500 (29.8172, 3.4908) -> (29.7296, 3.5867)
  line L501 (29.7296, 3.5867) -> (29.687, 3.6353)
  line L502 (29.687, 3.6353) -> (29.6453, 3.6844)
  line L503 (29.6453, 3.6844) -> (28.6812, 3.2158)
  line L504 (28.6812, 3.2158) -> (28.694, 3.1527)
  line L505 (28.694, 3.1527) -> (28.7059, 3.0892)
  line L506 (28.7059, 3.0892) -> (28.7272, 2.961)
  line L507 (28.7272, 2.961) -> (28.7607, 2.7009)
  line L508 (28.7607, 2.7009) -> (28.783, 2.4362)
  line L509 (28.783, 2.4362) -> (28.7951, 2.1675)
  line L510 (28.7951, 2.1675) -> (28.7976, 1.8951)
  line L511 (28.7976, 1.8951) -> (28.7909, 1.6195)
  line L512 (28.7909, 1.6195) -> (27.8707, 1.2585)
  line L513 (27.8707, 1.2585) -> (27.6783, 1.456)
  line L514 (27.6783, 1.456) -> (27.495, 1.6574)
  line L515 (27.495, 1.6574) -> (27.3211, 1.8627)
  line L516 (27.3211, 1.8627) -> (27.1575, 2.072)
  line L517 (27.1575, 2.072) -> (27.0052, 2.2855)
  line L518 (27.0052, 2.2855) -> (26.9337, 2.3939)
  line L519 (26.9337, 2.3939) -> (26.8992, 2.4486)
  line L520 (26.8992, 2.4486) -> (26.8656, 2.5036)
  line L521 (26.8656, 2.5036) -> (25.8401, 2.1916)
  line L522 (25.8401, 2.1916) -> (25.8429, 2.1273)
  line L523 (25.8429, 2.1273) -> (25.8447, 2.0627)
  line L524 (25.8447, 2.0627) -> (25.8457, 1.9328)
  line L525 (25.8457, 1.9328) -> (25.838, 1.6706)
  line L526 (25.838, 1.6706) -> (25.8187, 1.4057)
  line L527 (25.8187, 1.4057) -> (25.7886, 1.1383)
  line L528 (25.7886, 1.1383) -> (25.7485, 0.8689)
  line L529 (25.7485, 0.8689) -> (25.6987, 0.5977)
  line L530 (25.6987, 0.5977) -> (24.7333, 0.3851)
  line L531 (24.7333, 0.3851) -> (24.5743, 0.6103)
  line L532 (24.5743, 0.6103) -> (24.4247, 0.8379)
  line L533 (24.4247, 0.8379) -> (24.2851, 1.0679)
  line L534 (24.2851, 1.0679) -> (24.1562, 1.3002)
  line L535 (24.1562, 1.3002) -> (24.0391, 1.5349)
  line L536 (24.0391, 1.5349) -> (23.9855, 1.6532)
  line L537 (23.9855, 1.6532) -> (23.96, 1.7126)
  line L538 (23.96, 1.7126) -> (23.9354, 1.7721)
  line L539 (23.9354, 1.7721) -> (22.8738, 1.6244)
  line L540 (22.8738, 1.6244) -> (22.8664, 1.5604)
  line L541 (22.8664, 1.5604) -> (22.8581, 1.4964)
  line L542 (22.8581, 1.4964) -> (22.8388, 1.3679)
  line L543 (22.8388, 1.3679) -> (22.7902, 1.1102)
  line L544 (22.7902, 1.1102) -> (22.7297, 0.8515)
  line L545 (22.7297, 0.8515) -> (22.6581, 0.5922)
  line L546 (22.6581, 0.5922) -> (22.5763, 0.3324)
  line L547 (22.5763, 0.3324) -> (22.4848, 0.0723)
  line L548 (22.4848, 0.0723) -> (21.498, 0.0133)
  line L549 (21.498, 0.0133) -> (21.3761, 0.2607)
  line L550 (21.3761, 0.2607) -> (21.264, 0.5089)
  line L551 (21.264, 0.5089) -> (21.1621, 0.7578)
  line L552 (21.1621, 0.7578) -> (21.0711, 1.0074)
  line L553 (21.0711, 1.0074) -> (20.9922, 1.2576)
  line L554 (20.9922, 1.2576) -> (20.9577, 1.3828)
  line L555 (20.9577, 1.3828) -> (20.9418, 1.4454)
  line L556 (20.9418, 1.4454) -> (20.9269, 1.5081)
  line L557 (20.9269, 1.5081) -> (19.8552, 1.5283)
  line L558 (19.8552, 1.5283) -> (19.8379, 1.4663)
  line L559 (19.8379, 1.4663) -> (19.8197, 1.4042)
  line L560 (19.8197, 1.4042) -> (19.7805, 1.2804)
  line L561 (19.7805, 1.2804) -> (19.6922, 1.0334)
  line L562 (19.6922, 1.0334) -> (19.592, 0.7874)
  line L563 (19.592, 0.7874) -> (19.4807, 0.5425)
  line L564 (19.4807, 0.5425) -> (19.3593, 0.2987)
  line L565 (19.3593, 0.2987) -> (19.2282, 0.0561)
  line L566 (19.2282, 0.0561) -> (18.2444, 0.1522)
  line L567 (18.2444, 0.1522) -> (18.1627, 0.4156)
  line L568 (18.1627, 0.4156) -> (18.0907, 0.6783)
  line L569 (18.0907, 0.6783) -> (18.029, 0.9401)
  line L570 (18.029, 0.9401) -> (17.9782, 1.2009)
  line L571 (17.9782, 1.2009) -> (17.9394, 1.4603)
  line L572 (17.9394, 1.4603) -> (17.9249, 1.5894)
  line L573 (17.9249, 1.5894) -> (17.919, 1.6537)
  line L574 (17.919, 1.6537) -> (17.9141, 1.7179)
  line L575 (17.9141, 1.7179) -> (16.8588, 1.9056)
  line L576 (16.8588, 1.9056) -> (16.832, 1.847)
  line L577 (16.832, 1.847) -> (16.8043, 1.7886)
  line L578 (16.8043, 1.7886) -> (16.7462, 1.6724)
  line L579 (16.7462, 1.6724) -> (16.6204, 1.4423)
  line L580 (16.6204, 1.4423) -> (16.4828, 1.215)
  line L581 (16.4828, 1.215) -> (16.3347, 0.9905)
  line L582 (16.3347, 0.9905) -> (16.1766, 0.7687)
  line L583 (16.1766, 0.7687) -> (16.0091, 0.5496)
  line L584 (16.0091, 0.5496) -> (15.0525, 0.7984)
  line L585 (15.0525, 0.7984) -> (15.013, 1.0713)
  line L586 (15.013, 1.0713) -> (14.983, 1.342)
  line L587 (14.983, 1.342) -> (14.963, 1.6103)
  line L588 (14.963, 1.6103) -> (14.9537, 1.8758)
  line L589 (14.9537, 1.8758) -> (14.9559, 2.1381)
  line L590 (14.9559, 2.1381) -> (14.9618, 2.2678)
  line L591 (14.9618, 2.2678) -> (14.9661, 2.3323)
  line L592 (14.9661, 2.3323) -> (14.9712, 2.3965)
  line L593 (14.9712, 2.3965) -> (13.9582, 2.7469)
  line L594 (13.9582, 2.7469) -> (13.9226, 2.6932)
  line L595 (13.9226, 2.6932) -> (13.8861, 2.6399)
  line L596 (13.8861, 2.6399) -> (13.8106, 2.5342)
  line L597 (13.8106, 2.5342) -> (13.6503, 2.3266)
  line L598 (13.6503, 2.3266) -> (13.4789, 2.1236)
  line L599 (13.4789, 2.1236) -> (13.2974, 1.9251)
  line L600 (13.2974, 1.9251) -> (13.1066, 1.7307)
  line L601 (13.1066, 1.7307) -> (12.9069, 1.5406)
  line L602 (12.9069, 1.5406) -> (12.001, 1.936)
  line L603 (12.001, 1.936) -> (12.0046, 2.2117)
  line L604 (12.0046, 2.2117) -> (12.0174, 2.4838)
  line L605 (12.0174, 2.4838) -> (12.0396, 2.7519)
  line L606 (12.0396, 2.7519) -> (12.0719, 3.0155)
  line L607 (12.0719, 3.0155) -> (12.1152, 3.2742)
  line L608 (12.1152, 3.2742) -> (12.1413, 3.4015)
  line L609 (12.1413, 3.4015) -> (12.1556, 3.4645)
  line L610 (12.1556, 3.4645) -> (12.1707, 3.5271)
  line L611 (12.1707, 3.5271) -> (11.225, 4.0316)
  line L612 (11.225, 4.0316) -> (11.1814, 3.9842)
  line L613 (11.1814, 3.9842) -> (11.137, 3.9372)
  line L614 (11.137, 3.9372) -> (11.0459, 3.8447)
  line L615 (11.0459, 3.8447) -> (10.8551, 3.6647)
  line L616 (10.8551, 3.6647) -> (10.6541, 3.491)
  line L617 (10.6541, 3.491) -> (10.4438, 3.3233)
  line L618 (10.4438, 3.3233) -> (10.2249, 3.1612)
  line L619 (10.2249, 3.1612) -> (9.9979, 3.0046)
  line L620 (9.9979, 3.0046) -> (9.165, 3.5369)
  line L621 (9.165, 3.5369) -> (9.2118, 3.8086)
  line L622 (9.2118, 3.8086) -> (9.2669, 4.0753)
  line L623 (9.2669, 4.0753) -> (9.3308, 4.3367)
  line L624 (9.3308, 4.3367) -> (9.404, 4.592)
  line L625 (9.404, 4.592) -> (9.4871, 4.8408)
  line L626 (9.4871, 4.8408) -> (9.5328, 4.9624)
  line L627 (9.5328, 4.9624) -> (9.5568, 5.0224)
  line L628 (9.5568, 5.0224) -> (9.5816, 5.0819)
  line L629 (9.5816, 5.0819) -> (8.7264, 5.7281)
  line L630 (8.7264, 5.7281) -> (8.676, 5.6881)
  line L631 (8.676, 5.6881) -> (8.6248, 5.6486)
  line L632 (8.6248, 5.6486) -> (8.5203, 5.5715)
  line L633 (8.5203, 5.5715) -> (8.3037, 5.4236)
  line L634 (8.3037, 5.4236) -> (8.0779, 5.2835)
  line L635 (8.0779, 5.2835) -> (7.844, 5.1507)
  line L636 (7.844, 5.1507) -> (7.6025, 5.0248)
  line L637 (7.6025, 5.0248) -> (7.3538, 4.9057)
  line L638 (7.3538, 4.9057) -> (6.6144, 5.5617)
  line L639 (6.6144, 5.5617) -> (6.7031, 5.8228)
  line L640 (6.7031, 5.8228) -> (6.7993, 6.0776)
  line L641 (6.7993, 6.0776) -> (6.9033, 6.3257)
  line L642 (6.9033, 6.3257) -> (7.0155, 6.5665)
  line L643 (7.0155, 6.5665) -> (7.1365, 6.7992)
  line L644 (7.1365, 6.7992) -> (7.2007, 6.9121)
  line L645 (7.2007, 6.9121) -> (7.2337, 6.9677)
  line L646 (7.2337, 6.9677) -> (7.2675, 7.0225)
  line L647 (7.2675, 7.0225) -> (6.524, 7.7946)
  line L648 (6.524, 7.7946) -> (6.4679, 7.7629)
  line L649 (6.4679, 7.7629) -> (6.4111, 7.732)
  line L650 (6.4111, 7.732) -> (6.2959, 7.6721)
  line L651 (6.2959, 7.6721) -> (6.0588, 7.5599)
  line L652 (6.0588, 7.5599) -> (5.8139, 7.4569)
  line L653 (5.8139, 7.4569) -> (5.5621, 7.3623)
  line L654 (5.5621, 7.3623) -> (5.3038, 7.2758)
  line L655 (5.3038, 7.2758) -> (5.0396, 7.197)
  line L656 (5.0396, 7.197) -> (4.4119, 7.9606)
  line L657 (4.4119, 7.9606) -> (4.5404, 8.2046)
  line L658 (4.5404, 8.2046) -> (4.6752, 8.4413)
  line L659 (4.6752, 8.4413) -> (4.8167, 8.67)
  line L660 (4.8167, 8.67) -> (4.9652, 8.8903)
  line L661 (4.9652, 8.8903) -> (5.1212, 9.1012)
  line L662 (5.1212, 9.1012) -> (5.2022, 9.2027)
  line L663 (5.2022, 9.2027) -> (5.2436, 9.2524)
  line L664 (5.2436, 9.2524) -> (5.2855, 9.3013)
  line L665 (5.2855, 9.3013) -> (4.6719, 10.1802)
  line L666 (4.6719, 10.1802) -> (4.6116, 10.1577)
  line L667 (4.6116, 10.1577) -> (4.5507, 10.136)
  line L668 (4.5507, 10.136) -> (4.4275, 10.0949)
  line L669 (4.4275, 10.0949) -> (4.1758, 10.0212)
  line L670 (4.1758, 10.0212) -> (3.9178, 9.9577)
  line L671 (3.9178, 9.9577) -> (3.6543, 9.9037)
  line L672 (3.6543, 9.9037) -> (3.3857, 9.8586)
  line L673 (3.3857, 9.8586) -> (3.1123, 9.8221)
  line L674 (3.1123, 9.8221) -> (2.6118, 10.6745)
  line L675 (2.6118, 10.6745) -> (2.7769, 10.8954)
  line L676 (2.7769, 10.8954) -> (2.9471, 11.1081)
  line L677 (2.9471, 11.1081) -> (3.1227, 11.3119)
  line L678 (3.1227, 11.3119) -> (3.3038, 11.5062)
  line L679 (3.3038, 11.5062) -> (3.4908, 11.6901)
  line L680 (3.4908, 11.6901) -> (3.5867, 11.7777)
  line L681 (3.5867, 11.7777) -> (3.6353, 11.8203)
  line L682 (3.6353, 11.8203) -> (3.6844, 11.862)
  line L683 (3.6844, 11.862) -> (3.2159, 12.8261)
  line L684 (3.2159, 12.8261) -> (3.1527, 12.8133)
  line L685 (3.1527, 12.8133) -> (3.0892, 12.8014)
  line L686 (3.0892, 12.8014) -> (2.9611, 12.7801)
  line L687 (2.9611, 12.7801) -> (2.7009, 12.7467)
  line L688 (2.7009, 12.7467) -> (2.4362, 12.7243)
  line L689 (2.4362, 12.7243) -> (2.1675, 12.7122)
  line L690 (2.1675, 12.7122) -> (1.8951, 12.7097)
  line L691 (1.8951, 12.7097) -> (1.6195, 12.7164)
  line L692 (1.6195, 12.7164) -> (1.2585, 13.6367)
  line L693 (1.2585, 13.6367) -> (1.456, 13.829)
  line L694 (1.456, 13.829) -> (1.6574, 14.0124)
  line L695 (1.6574, 14.0124) -> (1.8627, 14.1862)
  line L696 (1.8627, 14.1862) -> (2.072, 14.3498)
  line L697 (2.072, 14.3498) -> (2.2855, 14.5022)
  line L698 (2.2855, 14.5022) -> (2.3939, 14.5737)
  line L699 (2.3939, 14.5737) -> (2.4486, 14.6082)
  line L700 (2.4486, 14.6082) -> (2.5036, 14.6417)
  line L701 (2.5036, 14.6417) -> (2.1916, 15.6672)
  line L702 (2.1916, 15.6672) -> (2.1273, 15.6645)
  line L703 (2.1273, 15.6645) -> (2.0627, 15.6626)
  line L704 (2.0627, 15.6626) -> (1.9328, 15.6616)
  line L705 (1.9328, 15.6616) -> (1.6706, 15.6693)
  line L706 (1.6706, 15.6693) -> (1.4057, 15.6886)
  line L707 (1.4057, 15.6886) -> (1.1383, 15.7187)
  line L708 (1.1383, 15.7187) -> (0.8689, 15.7589)
  line L709 (0.8689, 15.7589) -> (0.5977, 15.8086)
  line L710 (0.5977, 15.8086) -> (0.3851, 16.774)
  line L711 (0.3851, 16.774) -> (0.6103, 16.9331)
  line L712 (0.6103, 16.9331) -> (0.838, 17.0827)
  line L713 (0.838, 17.0827) -> (1.0679, 17.2223)
  line L714 (1.0679, 17.2223) -> (1.3002, 17.3511)
  line L715 (1.3002, 17.3511) -> (1.5349, 17.4682)
  line L716 (1.5349, 17.4682) -> (1.6532, 17.5219)
  line L717 (1.6532, 17.5219) -> (1.7126, 17.5474)
  line L718 (1.7126, 17.5474) -> (1.7722, 17.5719)
  line L719 (1.7722, 17.5719) -> (1.6245, 18.6336)
  circle A0 centre (20.7537, 20.7537) radius 0.5
  point P0 (0, 0)
  constraints: 1440 end point, 358 perpendicular, 169 parallel, 1 centre point
extrude "Extrusion2" add sketch "Sketch5" along normal blind 5
sketch "Sketch6" plane through (0, 0, 0) normal (0, -1, 0) x (1, 0, 0)
  circle A0 centre (-20.7537, 20.7537) radius 0.5 construction
  circle A1 centre (-20.7537, 20.7537) radius 15
  point P0 (0, 0)
  dimension "d6" = 30
  constraints: 1 centre point, 1 coincident
  measures "d6" diameter of A1
extrude "Extrusion3" [suppressed]
sketch "Sketch7" plane through (-20.7537, -2.5, 20.7537) normal (0, -1, 0) x (1, 0, 0)
  circle A0 centre (0, 0) radius 15 construction
  line L0 (-0.1414, -2.1213) -> (-2.1213, -0.1414)
  line L1 (-2.1213, 0.1414) -> (-0.1414, 2.1213)
  line L2 (0.1414, 2.1213) -> (2.1213, 0.1414)
  line L3 (2.1213, -0.1414) -> (0.1414, -2.1213)
  line L4 (0, -2.2627) -> (0, 2.2627) construction
  line L5 (-2.2627, 0) -> (2.2627, 0) construction
  arc A1 (-2.1213, 0.1414) -> (-2.1213, -0.1414) centre (-1.9799, 0) ccw
  arc A2 (-0.1414, -2.1213) -> (0.1414, -2.1213) centre (0, -1.9799) ccw
  arc A3 (2.1213, -0.1414) -> (2.1213, 0.1414) centre (1.9799, 0) ccw
  arc A4 (0.1414, 2.1213) -> (-0.1414, 2.1213) centre (0, 1.9799) ccw
  circle A5 centre (10, 0) radius 2.45
  circle A6 centre (-10, 0) radius 2.45
  circle A7 centre (0, -10) radius 2.45
  circle A8 centre (0, 10) radius 2.45
  point P0 (20.7537, -20.7537)
  dimension "d9" = 3.2
  dimension "d10" = 3.2
  dimension "d11" = 0.2
  dimension "d12" = 4.9
  dimension "d13" = 4.9
  dimension "d14" = 4.9
  dimension "d15" = 4.9
  dimension "d16" = 20
  dimension "d17" = 10
  dimension "d18" = 20
  dimension "d19" = 10
  constraints: 12 end point, 12 point on line, 8 centre point, 8 point on circle, 8 tangent, 3 equal radius, 2 midpoint, 2 parallel, 1 horizontal, 1 perpendicular
  measures "d9" distance of L4.end L5.end
  measures "d10" distance of L5.start L4.end
  measures "d11" radius of A1
  measures "d12" diameter of A5
  measures "d13" diameter of A6
  measures "d14" diameter of A7
  measures "d15" diameter of A8
  measures "d16" distance of A7.centre A8.centre
  measures "d17" distance from line of L5 A7.centre
  measures "d18" distance of A5.centre A6.centre
  measures "d19" distance of A0.centre A6.centre
extrude "Extrusion4" [suppressed]
sketch "Sketch9" plane through (0, 5, 0) normal (0, 1, 0) x (1, 0, 0)
  circle A0 centre (-11.0757, -23.271) radius 2.45 projected
  circle A1 centre (-30.4316, -18.2364) radius 2.45 projected
  arc A2 (-21.4245, -22.7711) -> (-21.1508, -22.8423) centre (-21.2521, -22.6698) ccw projected
  line L0 (-21.1508, -22.8423) -> (-18.7363, -21.4245) projected
  arc A3 (-18.7363, -21.4245) -> (-18.6651, -21.1508) centre (-18.8375, -21.2521) ccw projected
  line L1 (-18.6651, -21.1508) -> (-20.0828, -18.7363) projected
  arc A4 (-20.0828, -18.7363) -> (-20.3565, -18.6651) centre (-20.2553, -18.8375) ccw projected
  line L2 (-20.3565, -18.6651) -> (-22.7711, -20.0828) projected
  arc A5 (-22.7711, -20.0828) -> (-22.8423, -20.3565) centre (-22.6698, -20.2553) ccw projected
  line L3 (-22.8423, -20.3565) -> (-21.4245, -22.7711) projected
  circle A6 centre (-18.2364, -11.0757) radius 2.45 projected
  circle A7 centre (-23.271, -30.4316) radius 2.45 projected
  circle A8 centre (-20.7537, -20.7537) radius 15 projected
  point P0 (0, 0)
extrude "Extrusion6" cut sketch "Sketch9" against normal through all contours A0 | A1 | L3 A5 L2 A4 L1 A3 L0 A2 | A6 | A7
equation "\"d10\" = d9"
equation "\"d13\" = d12"
equation "\"d14\" = d12"
equation "\"d15\" = d12"
equation "\"d17\" = 0.5 * d16"
equation "\"d18\" = d16"
equation "\"d19\" = 0.5 * d18"
body "Solid2"
